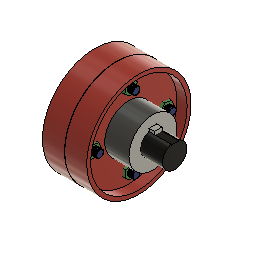
flange joint (Autodesk Fusion 360 design; units mm, degrees)
Autodesk Fusion 360 part; units mm, degrees
sketch "Sketch1" plane through (0, 0, 0) normal (0, 1, 0) x (1, 0, 0)
  line L0 (-10, -25) -> (-90, -25)
  line L1 (16, -25) -> (85, -25)
  line L2 (95, 0) -> (-100, 0) construction
  line L3 (-10, -25) -> (-10, -37.5)
  line L4 (-10, -37.5) -> (-15, -37.5)
  line L5 (-15, -37.5) -> (-15, -108)
  line L6 (-15, -108) -> (-61, -108)
  line L7 (-61, -108) -> (-61, -100)
  line L8 (-61, -100) -> (-40, -100)
  line L9 (-90, -25) -> (-90, -50)
  line L10 (-90, -50) -> (-40, -50)
  line L11 (-40, -50) -> (-40, -100)
  line L12 (16, -25) -> (16, -37.5)
  line L13 (16, -37.5) -> (10, -37.5)
  line L14 (10, -37.5) -> (10, -107.5)
  line L15 (10, -107.5) -> (56, -107.5)
  line L16 (56, -107.5) -> (56, -99.5)
  line L17 (56, -99.5) -> (35, -99.5)
  line L18 (35, -99.5) -> (35, -49.5)
  line L19 (35, -49.5) -> (85, -49.5)
  line L20 (85, -25) -> (85, -49.5)
  dimension "d7" = 12.5
  dimension "d8" = 5
  dimension "d10" = 46
  dimension "d11" = 8
  dimension "d12" = 21
  dimension "d14" = 70.5
  dimension "d15" = 108
  dimension "d16" = 80
  dimension "d17" = 25
  dimension "d18" = 50
  dimension "d19" = 50
  dimension "d21" = 12.5
  dimension "d22" = 6
  dimension "d23" = 70
  dimension "d24" = 25
  dimension "d25" = 46
  dimension "d26" = 8
  dimension "d27" = 21
  dimension "d28" = 50
  constraint horizontal L2
  constraint perpendicular L0 L3
  constraint perpendicular L3 L4
  constraint perpendicular L4 L5
  constraint perpendicular L5 L6
  constraint perpendicular L6 L7
  constraint perpendicular L7 L8
  constraint perpendicular L0 L9
  constraint perpendicular L9 L10
  constraint perpendicular L1 L12
  constraint perpendicular L12 L13
  constraint perpendicular L13 L14
  constraint perpendicular L14 L15
  constraint perpendicular L15 L16
  constraint perpendicular L16 L17
  constraint perpendicular L17 L18
  constraint perpendicular L18 L19
  constraint perpendicular L19 L20
  measures "d7" distance of L0.start L3.end
  measures "d8" distance of L3.end L4.end
  measures "d10" distance of L5.end L6.end
  measures "d11" distance of L6.end L7.end
  measures "d12" distance of L7.end L8.end
  measures "d14" distance of L4.end L5.end
  measures "d15" vertical distance of origin L5.end
  measures "d16" distance of L0.start L0.end
  measures "d17" distance of L0.end L9.end
  measures "d18" distance of L9.end L10.end
  measures "d19" distance of L8.end L10.end
  measures "d21" distance of L1.start L12.end
  measures "d22" distance of L12.end L13.end
  measures "d23" distance of L13.end L14.end
  measures "d24" horizontal distance of L5.end L14.end
  measures "d25" distance of L14.end L15.end
  measures "d26" distance of L15.end L16.end
  measures "d27" distance of L16.end L17.end
  measures "d28" distance of L17.end L18.end
revolve "Revolve1" add sketch "Sketch1" angle 360 about axis through (95, 0, 0) along (-1, 0, 0) makes body 1 at (-15, -5.3655, 84.0979) makes body 2 at (10, -5.3407, 83.7664)
sketch "Sketch2" plane through (0, 0, 0) normal (1, 0, 0) x (0, 1, 0)
  line L0 (0, 0) -> (0, 19)
  line L1 (0, 19) -> (8, 19)
  line L2 (8, 19) -> (8, 29)
  line L3 (8, 29) -> (-8, 29)
  line L4 (-8, 29) -> (-8, 19)
  line L5 (-8, 19) -> (0, 19)
  dimension "d31" = 8
  dimension "d32" = 10
  dimension "d33" = 16
  dimension "d34" = 10
  constraint coincident L0.start origin
  constraint vertical L0
  constraint perpendicular L0 L1
  constraint perpendicular L1 L2
  constraint perpendicular L2 L3
  constraint perpendicular L3 L4
  measures "d31" distance of L0.end L1.end
  measures "d32" distance of L1.end L2.end
  measures "d33" distance of L2.end L3.end
  measures "d34" distance of L3.end L4.end
extrude "Extrude1" cut sketch "Sketch2" along normal blind 85 and the other way blind 90 bodies 1 2
sketch "Sketch3" plane through (-15, 0, 0) normal (1, 0, 0) x (0, 1, 0)
  circle A0 centre (0, 0) radius 37.5
  circle A1 centre (0, 0) radius 108
  circle A2 centre (0, 75) radius 8
  circle A3 centre (-75, 0) radius 8
  circle A4 centre (0, -75) radius 8
  circle A5 centre (75, 0) radius 8
  dimension "d40" = 16
  dimension "d42" = 360
  measures "d40" diameter of A2
extrude "Extrude2" cut sketch "Sketch3" along normal blind 100 and the other way blind 75 contours A2 | A3 | A4 | A5 bodies 1 2
sketch "Sketch4" plane through (0, 0, 0) normal (0, 0, 1) x (1, 0, 0)
  line L0 (12.919, -5.01) -> (10.7983, 8.6831)
  line L1 (10.7983, 8.6831) -> (-2.1207, 13.6932)
  line L2 (-2.1207, 13.6932) -> (-12.919, 5.01)
  line L3 (-12.919, 5.01) -> (-10.7983, -8.6831)
  line L4 (-10.7983, -8.6831) -> (2.1207, -13.6932)
  line L5 (2.1207, -13.6932) -> (12.919, -5.01)
  circle A0 centre (0, 0) radius 8
  dimension "d47" = 12
  dimension "d48" = 16
  constraint coincident A0.centre origin
  measures "d47" distance of A0.centre L5
  measures "d48" diameter of A0
extrude "Extrude3" add sketch "Sketch4" along normal blind 12 separate body contours L0 L1 L2 L3 L4 L5 | A0 makes body 3
extrude "Extrude4" add sketch "Sketch4" against normal blind 66 contours A0 bodies 3
sketch "Sketch5" plane through (0, 0, 0) normal (0, 0, 1) x (1, 0, 0)
  line L0 (51.672, -7.4676) -> (52.3031, 6.3744)
  line L1 (52.3031, 6.3744) -> (40.6311, 13.842)
  line L2 (40.6311, 13.842) -> (28.328, 7.4676)
  line L3 (28.328, 7.4676) -> (27.6969, -6.3744)
  line L4 (27.6969, -6.3744) -> (39.3689, -13.842)
  line L5 (39.3689, -13.842) -> (51.672, -7.4676)
  circle A0 centre (40, 0) radius 8
  point P0 (40, 0)
  dimension "d53" = 12
  dimension "d54" = 16
  constraint coincident P0 A0.centre
  measures "d53" distance of P0 L5
  measures "d54" diameter of A0
extrude "Extrude5" add sketch "Sketch5" along normal blind 14 separate body makes body 4
thread "Thread1" "ISO Metric profile 16.0 M16x2 6g" major diameter 15.822 minor diameter 13.534 pitch 2 angle 60 modelled right hand crest width 0.2847 on face at (7.9602, -0.7965, -44) from (0, 0, -41) to (0, 0, -66) crest through (7.911, 0, 0.5) on bodies 3
thread "Thread2" "ISO Metric profile 16.0 M16x2 6H" major diameter 16.2505 minor diameter 14.0225 pitch 2 angle 60 modelled right hand crest width 0.5471 on face at (47.9602, -0.7965, 9.3333) crest through (47.0113, 0, 0.5) on bodies 4
sketch "Sketch6" plane through (0, 0, 0) normal (0, 1, 0) x (1, 0, 0)
  line L0 (8, 5) -> (-8, 5)
  line L1 (-8, 5) -> (-8, -5)
  line L2 (-8, -5) -> (8, -5)
  line L3 (8, -5) -> (8, 5)
  line L4 (8, 5) -> (-8, -5) construction
  line L5 (-8, 5) -> (8, -5) construction
  dimension "d61" = 16
  dimension "d62" = 10
  constraint horizontal L0
  constraint perpendicular L0 L1
  constraint parallel L0 L2
  constraint parallel L1 L3
  constraint coincident L4 origin
  constraint coincident L5 origin
  measures "d61" distance of L1.end L2.end
  measures "d62" distance of L0.end L1.end
ref_plane "WorkPlane1" through (0, 85, 0) normal (0, 1, 0) x (1, 0, 0)
sketch "Sketch7" plane through (0, 85, 0) normal (0, 1, 0) x (1, 0, 0)
  line L0 (-7.95, 4.95) -> (7.95, 4.95)
  line L1 (7.95, 4.95) -> (7.95, -4.95)
  line L2 (7.95, -4.95) -> (-7.95, -4.95)
  line L3 (-7.95, -4.95) -> (-7.95, 4.95)
  line L4 (-7.95, 4.95) -> (7.95, -4.95) construction
  line L5 (7.95, 4.95) -> (-7.95, -4.95) construction
  dimension "d64" = 15.9
  dimension "d65" = 9.9
  constraint horizontal L0
  constraint perpendicular L0 L1
  constraint parallel L0 L2
  constraint parallel L1 L3
  constraint coincident L4 origin
  constraint coincident L5 origin
  measures "d64" distance of L1.end L2.end
  measures "d65" distance of L0.end L1.end
loft "Loft1" add profiles "Sketch7", "Sketch6" section 1 section 2 separate body makes body 5
sketch "Sketch8" plane through (0, 0, 0) normal (1, 0, 0) x (0, 1, 0)
  circle A0 centre (0, 0) radius 25
  dimension "d66" = 50
  constraint coincident A0.centre origin
  measures "d66" diameter of A0
extrude "Extrude6" add sketch "Sketch8" along normal blind 110 separate body makes body 6
sketch "Sketch9" plane through (0, 0, 0) normal (-1, 0, 0) x (0, -1, 0)
  circle A0 centre (0, 0) radius 25
  line L0 (0, 19) -> (8, 19)
  line L1 (0, 19) -> (-8, 19)
  line L2 (0, 25) -> (8, 25)
  line L3 (8, 25) -> (8, 19)
  line L4 (0, 25) -> (-8, 25)
  line L5 (-8, 25) -> (-8, 19)
  dimension "d69" = 6
  dimension "d70" = 8
  dimension "d71" = 8
  constraint coincident A0 L2.start
  constraint perpendicular L2 L3
  constraint perpendicular L1 L5
  measures "d69" distance of L2.start L0.start
  measures "d70" distance of L0.start L0.end
  measures "d71" distance of L0.start L1.end
sketch "Sketch12" plane through (0, 0, 0) normal (-1, 0, 0) x (0, -1, 0)
  circle A0 centre (0, 0) radius 25
  line L0 (-0.7321, -24.9893) -> (-0.7321, -30.9893)
  line L1 (-0.7321, -30.9893) -> (-8.7321, -30.9893)
  line L2 (-0.7321, -30.9893) -> (7.2679, -30.9893)
  line L3 (-8.7321, -30.9893) -> (-8.7321, -22.055)
  line L4 (-8.7321, -22.055) -> (7.393, -22.055)
  line L5 (7.393, -22.055) -> (7.2679, -30.9893)
  dimension "d91" = 6
  dimension "d92" = 8
  dimension "d93" = 8
  constraint coincident A0 L0.start
  constraint vertical L0
  constraint perpendicular L0 L1
  constraint perpendicular L0 L2
  constraint perpendicular L1 L3
  constraint perpendicular L3 L4
  measures "d91" distance of L0.start L0.end
  measures "d92" distance of L0.end L1.end
  measures "d93" distance of L0.end L2.end
extrude "Extrude8" cut sketch "Sketch12" against normal blind 90 contours A0 L3 L4 L5 | A0 L0 L1 L3 | A0 L0 L2 L5 picked at (-1.5965, -22.9569) bodies 6
copy_body "Body->Comp1" bodies 1 removing the originals makes body 7 in component "Flange A"
copy_body "Body->Comp2" bodies 2 removing the originals makes body 8 in component "Flange B"
copy_body "Body->Comp3" bodies 3 removing the originals makes body 9 in component "bolt"
copy_body "Body->Comp4" bodies 4 removing the originals makes body 10 in component "nut"
copy_body "Body->Comp5" bodies 5 removing the originals makes body 11 in component "taper key"
copy_body "Body->Comp6" bodies 6 removing the originals makes body 12 in component "shaft"
move_body "Move1" bodies 11 to x (0, -1, -0.000589) y (1, 0, -0.000588) z (0.000588, -0.000589, 1) at (-50.475, 21.8828, -5.9057) in component "taper key"
move_body "Move1'" bodies 12 to x (1, 0, 0) y (0, 1, 0) z (0, 0, 1) at (0, 50.5, 18.9) in component "shaft"
move_body "Move2" bodies 11 to x (1, 0, 0) y (0, 1, 0) z (0, 0, 1) at (104.9981, 1.0624, -1.1229) in component "taper key"
sketch "Sketch10" plane through (-121.7563, 0, 0) normal (1, 0, 0) x (0, 1, 0)
  circle A0 centre (7.1202, -1.8417) radius 25
  circle A1 centre (7.1202, -1.8417) radius 0.5
  dimension "d86" = 1
  constraint concentric A0 A1
  measures "d86" diameter of A1
sketch "Sketch13" plane through (0, 0, 0) normal (0, 1, 0) x (1, 0, 0)
  line L0 (16, -37.5) -> (10, -37.5)
  line L1 (-10, -37.5) -> (-15, -37.5)
  dimension "d104" = 6
  dimension "d105" = 5
  measures "d104" distance of L0.start L0.end
  measures "d105" distance of L1.start L1.end
move_body "Move3" bodies 11 to x (1, 0, 0) y (0, 1, 0) z (0, 0, 1) at (0, 90, 0.053) in component "taper key"
move_body "Move2'" bodies 12 to x (1, 0, 0) y (0, 1, 0) z (0, 0, 1) at (90, 0, 0) in component "shaft"
move_body "Move1''" bodies 9 to x (1, 0, 0) y (0, 1, 0) z (0, 0, 1) at (0, -10, 0) in component "bolt"
move_body "Move1'''" bodies 10 to x (1, 0, 0) y (0, 1, 0) z (0, 0, 1) at (0.8716, -9.9619, 0) in component "nut"
move_body "Move4" bodies 11 to x (1, 0, 0) y (0, 1, 0) z (0, 0, 1) at (0, -10, -0.0059) in component "taper key"
move_body "Move1''''" bodies 7 to x (1, 0, 0) y (0, 1, 0) z (0, 0, 1) at (0, -10, 0) in component "Flange A"
move_body "Move1'''''" bodies 8 to x (1, 0, 0) y (0, 1, 0) z (0, 0, 1) at (0, -10, 0) in component "Flange B"
move_body "Move3'" bodies 12 to x (1, 0, 0) y (0, 1, 0) z (0, 0, 1) at (0, 0, -10) in component "shaft"
move_body "Move4'" bodies 12 to x (1, 0, 0) y (0, 0, 1) z (0, -1, 0) at (-100, 57.8552, -42.8012) in component "shaft"
move_body "Move5" bodies 12 to x (1, 0, 0) y (0, 0, 1) z (0, -1, 0) at (-185, 48.9358, -30.6078) in component "shaft"
move_body "Move5'" bodies 11 to x (1, 0, 0) y (0, 1, 0) z (0, 0, 1) at (-175.0117, -99.9883, -19.956) in component "taper key"
component_pattern "component pattern"
move_body "Move6" bodies 12 to x (-1, 0, 0) y (0, -1, 0) z (0, 0, 1) at (-160, 66.4581, 0) in component "shaft"
move_body "Move7" bodies 12 to x (1, 0, 0) y (0, 1, 0) z (0, 0, 1) at (0, 15, 0) in component "shaft"
component "Flange A" placed x (1, 0, 0) y (0, 1, 0) z (0, 0, 1) at (-98.6182, 7.1518, -1.7034)
component "Flange B" placed x (1, 0, 0) y (0, 1, 0) z (0, 0, 1) at (-124.6182, 7.1518, -1.6462)
component "bolt" placed x (0, 0, 1) y (0, 1, 0) z (-1, 0, 0) at (-139.6182, 82.383, -1.7028)
component "nut" placed x (0, -0.087156, -0.996195) y (0, 0.996195, -0.087156) z (1, 0, 0) at (-98.6182, 85.7357, 38.4552)
component "taper key" placed x (1, 0, 0) y (0, 1, -0.000589) z (0, 0.000589, 1) at (6.8675, -5.7893, 49.3357)
component "shaft" placed x (1, 0, 0) y (0, 1, 0) z (0, 0, 1) at (-28.6182, -44.0852, -20.0509)
component "bolt" placed x (0, -1, 0) y (0, 0, 1) z (-1, 0, 0) at (-139.6182, -2.8488, 83.5277)
component "nut" placed x (0, 0.996195, -0.087156) y (0, 0.087156, 0.996195) z (1, 0, 0) at (-98.6182, -43.0068, 86.8805)
component "bolt" placed x (0, 0, -1) y (0, -1, 0) z (-1, 0, 0) at (-139.6182, -88.0793, -1.704)
component "nut" placed x (0, 0.087156, 0.996195) y (0, -0.996195, 0.087156) z (1, 0, 0) at (-98.6182, -91.4321, -41.8621)
component "bolt" placed x (0, 1, 0) y (0, 0, -1) z (-1, 0, 0) at (-139.6182, -2.8476, -86.9346)
component "nut" placed x (0, -0.996195, 0.087156) y (0, -0.087156, -0.996195) z (1, 0, 0) at (-98.6182, 37.3104, -90.2874)
equation "d64 = 16 mm - 0.1 mm"
equation "d65 = 10 mm - 0.1 mm"
named bodies: "Flange A", "Flange B", "bolt", "nut", "taper key", "shaft"
